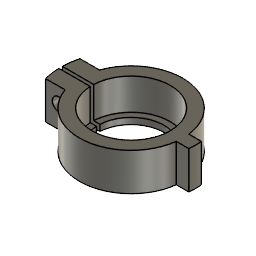
Lenshouder binnen (Autodesk Fusion 360 design; units mm, degrees)
part number: 2026-06-04-12-54-56-357
Autodesk Fusion 360 part; units mm, degrees
sketch "Main ring profile" plane through (0, 0, 0) normal (0, 0, 1) x (1, 0, 0)
  circle A0 centre (0, 0) radius 12.5
  dimension "d1" = 25
  constraint coincident A0.centre origin
  measures "d1" diameter of A0
extrude "Extrude1" add sketch "Main ring profile" along normal blind 2 thin wall 2 inside
extrude "Extrude2" add sketch "Main ring profile" along normal blind 12 thin wall 4 outside
sketch "Middle ring profile" plane through (0, 0, 0) normal (0, 0, 1) x (1, 0, 0)
  circle A0 centre (0, 0) radius 20.5
  line L0 (15.5, -2) -> (21.5, -2)
  line L1 (21.5, -2) -> (21.5, 2)
  line L2 (21.5, 2) -> (15.5, 2)
  line L3 (15.5, 2) -> (15.5, -2)
  line L4 (15.5, -2) -> (21.5, 2) construction
  line L5 (21.5, -2) -> (15.5, 2) construction
  point P0 (18.5, 0)
  dimension "d8" = 41
  dimension "d9" = 6
  dimension "d10" = 4
  dimension "d11" = 21.5
  dimension "d12" = 2
  constraint coincident A0.centre origin
  constraint horizontal L0
  constraint perpendicular L0 L1
  constraint parallel L0 L2
  constraint parallel L1 L3
  constraint coincident L4 P0
  constraint coincident L5 P0
  measures "d8" diameter of A0
  measures "d9" distance of L1.end L2.end
  measures "d10" distance of L0.end L1.end
  measures "d11" distance of A0.centre L1
  measures "d12" distance of A0.centre L0
extrude "Extrude3" add sketch "Middle ring profile" along normal blind 12 contours A0 L0 L2 L3 picked at (17.1667, 0)
sketch "Outer ring profile" plane through (0, 0, 0) normal (0, 0, 1) x (1, 0, 0)
  circle A0 centre (0, 0) radius 22.5
  line L0 (-24, -5.5) -> (-15, -5.5)
  line L1 (-15, -5.5) -> (-15, 5.5)
  line L2 (-15, 5.5) -> (-24, 5.5)
  line L3 (-24, 5.5) -> (-24, -5.5)
  line L4 (-24, -5.5) -> (-15, 5.5) construction
  line L5 (-15, -5.5) -> (-24, 5.5) construction
  point P0 (-19.5, 0)
  dimension "d15" = 45
  dimension "d16" = 9
  dimension "d17" = 11
  dimension "d18" = 24
  dimension "d19" = 5.5
  constraint coincident A0.centre origin
  constraint horizontal L0
  constraint perpendicular L0 L1
  constraint parallel L0 L2
  constraint parallel L1 L3
  constraint coincident L4 P0
  constraint coincident L5 P0
  measures "d15" diameter of A0
  measures "d16" distance of L1.end L2.end
  measures "d17" distance of L0.end L1.end
  measures "d18" distance of A0.centre L3
  measures "d19" distance of A0.centre L0
extrude "Extrude4" add sketch "Outer ring profile" along normal blind 12 contours A0 L0 L1 L2 picked at (-17.5, 0)
sketch "Cutout profile" plane through (0, 0, 0) normal (0, 0, 1) x (1, 0, 0)
  line L0 (0, 0.55) -> (-30, 0.55)
  line L1 (-30, 0.55) -> (-30, -0.55)
  line L2 (-30, -0.55) -> (0, -0.55)
  line L3 (0, -0.55) -> (0, 0.55)
  line L4 (0, 0.55) -> (-30, -0.55) construction
  line L5 (-30, 0.55) -> (0, -0.55) construction
  line L6 (0, 1.75) -> (0, 22.5)
  line L7 (1.75, 0) -> (22.5, 0)
  point P0 (-15, 0)
  dimension "d22" = 30
  dimension "d23" = 1.1
  dimension "d24" = 0.55
  constraint horizontal L0
  constraint perpendicular L0 L1
  constraint parallel L0 L2
  constraint parallel L1 L3
  constraint coincident L4 P0
  constraint coincident L5 P0
  constraint collinear L3 L6
  measures "d22" distance of L1.end L2.end
  measures "d23" distance of L0.end L1.end
  measures "d24" distance of L2 L7
extrude "Extrude5" cut sketch "Cutout profile" along normal blind 12
ref_plane "WorkPlane2" through (0, 0, 7) normal (0, 0, 1) x (1, 0, 0)
sketch "Screw hole profile" plane through (0, 5.5, 0) normal (0, 1, 0) x (-1, 0, 0)
  line L0 (15.5563, 12) -> (15.5563, 0)
  line L1 (15.5563, 0) -> (21.8174, 0)
  line L2 (21.8174, 0) -> (21.8174, 12)
  line L3 (21.8174, 12) -> (15.5563, 12)
  line L4 (15.5563, 6) -> (21.8174, 6) construction
  line L5 (20.8516, 7) -> (-19.4011, 7) construction
  line L6 (15.5563, 7) -> (21.8174, 7) construction
  circle A0 centre (17.5174, 7) radius 2.75
  circle A1 centre (17.5174, 7) radius 1.5
  dimension "d35" = 5.5
  dimension "d36" = 3
  dimension "d43" = 4.3
  constraint midpoint L0 L4.start
  constraint midpoint L2 L4.end
  constraint coincident L5 L6.start
  constraint coincident L0 L6.start
  constraint coincident L2 L6.end
  constraint perpendicular L2 L6
  constraint coincident L6 A0.centre
  constraint concentric A0 A1
  measures "d35" diameter of A0
  measures "d36" diameter of A1
  measures "d43" distance of L2 A0.centre
extrude "Extrude6" cut sketch "Screw hole profile" against normal blind 11 contours A1
extrude "Extrude7" cut sketch "Screw hole profile" along normal mid plane 6 contours L0 A0 | L0 A0
sketch "Threaded insert hole" plane through (0, -5.5, 0) normal (0, -1, 0) x (1, 0, 0)
  circle A0 centre (-17.5174, 7) radius 1.5
  line L0 (-15.5563, 0) -> (-15.5563, 12)
  line L1 (-15.5563, 12) -> (-21.8174, 12)
  line L2 (-21.8174, 12) -> (-21.8174, 0)
  line L3 (-21.8174, 0) -> (-15.5563, 0)
  circle A1 centre (-17.5174, 7) radius 2.1
  dimension "d37" = 4.2
  constraint concentric A0 A1
  measures "d37" diameter of A1
extrude "Extrude8" cut sketch "Threaded insert hole" along normal blind 10 and the other way blind 5.5 contours L0 A1 | L0 A1
scale "Scale1" factor 1.008 about (-15.5563, 5.5, 0) bodies 1
equation "d24 = d23 / 2"
